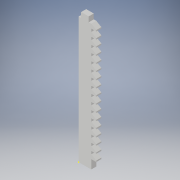
# Autodesk Inventor part: graduated_foot
Saved by Autodesk Inventor 2019.4 (Build 234330000, 330)
## iProperties
Created: 2019-12-14
Part Number: graduated_foot
Material: Generic
Document SubType Name: Modeling
Designer: fabfarm
Density: 1 g/cm^3
Appearance: Default
Author: fabfarm
Autodesk Inventor part; units mm, degrees
ref_plane "YZ Plane" through (0, 0, 0) normal (1, 0, 0) x (0, 1, 0)
ref_plane "XZ Plane" through (0, 0, 0) normal (0, 1, 0) x (-1, 0, 0)
ref_plane "XY Plane" through (0, 0, 0) normal (0, 0, 1) x (1, 0, 0)
sketch "Sketch4" plane through (0, 0, 0) normal (0, 0, 1) x (1, 0, 0)
  line L0 (0, 500) -> (50, 500)
  line L1 (50, 500) -> (50, 0)
  line L2 (50, 0) -> (0, 0)
  line L3 (0, 0) -> (0, 500)
  dimension "d31" = 50
  dimension "d32" = 500
  constraints: 8 end point, 2 parallel, 2 point on line, 1 horizontal, 1 perpendicular
  measures "d31" distance of L0.start L0.end
  measures "d32" distance of L2.end L0.start
extrude "Extrusion1" add sketch "Sketch4" along normal blind 20.18
sketch "Sketch5" plane through (0, 0, 20.18) normal (0, 0, 1) x (1, 0, 0)
  line L0 (50, 500) -> (0, 500) projected
  line L1 (10, 500) -> (40, 500)
  line L2 (40, 500) -> (40, 520.18)
  line L3 (40, 520.18) -> (10, 520.18)
  line L4 (10, 520.18) -> (10, 500)
  line L5 (0, 500) -> (0, 0) projected
  line L6 (50, 0) -> (50, 500) projected
  dimension "d46" = 10
  dimension "d47" = 10
  dimension "d48" = 20.18
  constraints: 8 end point, 2 parallel, 1 horizontal, 1 perpendicular, 1 point on line
  measures "d46" distance between parallel lines of L5 L4
  measures "d47" distance between parallel lines of L6 L2
  measures "d48" distance of L3.end L1.start
extrude "Extrusion2" add sketch "Sketch5" against normal blind 20.18
sketch "Sketch6" plane through (0, 0, 20.18) normal (0, 0, 1) x (1, 0, 0)
  line L0 (50, 500) -> (70, 488.453)
  line L1 (70, 488.453) -> (70, 483.453)
  line L2 (70, 483.453) -> (50, 483.453)
  line L3 (50, 500) -> (40, 500) projected
  line L4 (40, 500) -> (50, 500) projected
  line L5 (50, 500) -> (50, 483.453)
  line L6 (50, 0) -> (50, 500) projected
  line L7 (50, 472) -> (70, 460.453)
  line L8 (70, 460.453) -> (70, 455.453)
  line L9 (70, 455.453) -> (50, 455.453)
  line L10 (50, 472) -> (50, 455.453)
  line L11 (50, 444) -> (70, 432.453)
  line L12 (70, 432.453) -> (70, 427.453)
  line L13 (70, 427.453) -> (50, 427.453)
  line L14 (50, 444) -> (50, 427.453)
  line L15 (50, 416) -> (70, 404.453)
  line L16 (70, 404.453) -> (70, 399.453)
  line L17 (70, 399.453) -> (50, 399.453)
  line L18 (50, 416) -> (50, 399.453)
  line L19 (50, 388) -> (70, 376.453)
  line L20 (70, 376.453) -> (70, 371.453)
  line L21 (70, 371.453) -> (50, 371.453)
  line L22 (50, 388) -> (50, 371.453)
  line L23 (50, 360) -> (70, 348.453)
  line L24 (70, 348.453) -> (70, 343.453)
  line L25 (70, 343.453) -> (50, 343.453)
  line L26 (50, 360) -> (50, 343.453)
  line L27 (50, 332) -> (70, 320.453)
  line L28 (70, 320.453) -> (70, 315.453)
  line L29 (70, 315.453) -> (50, 315.453)
  line L30 (50, 332) -> (50, 315.453)
  line L31 (50, 304) -> (70, 292.453)
  line L32 (70, 292.453) -> (70, 287.453)
  line L33 (70, 287.453) -> (50, 287.453)
  line L34 (50, 304) -> (50, 287.453)
  line L35 (50, 276) -> (70, 264.453)
  line L36 (70, 264.453) -> (70, 259.453)
  line L37 (70, 259.453) -> (50, 259.453)
  line L38 (50, 276) -> (50, 259.453)
  line L39 (50, 248) -> (70, 236.453)
  line L40 (70, 236.453) -> (70, 231.453)
  line L41 (70, 231.453) -> (50, 231.453)
  line L42 (50, 248) -> (50, 231.453)
  line L43 (50, 220) -> (70, 208.453)
  line L44 (70, 208.453) -> (70, 203.453)
  line L45 (70, 203.453) -> (50, 203.453)
  line L46 (50, 220) -> (50, 203.453)
  line L47 (50, 192) -> (70, 180.453)
  line L48 (70, 180.453) -> (70, 175.453)
  line L49 (70, 175.453) -> (50, 175.453)
  line L50 (50, 192) -> (50, 175.453)
  line L51 (50, 164) -> (70, 152.453)
  line L52 (70, 152.453) -> (70, 147.453)
  line L53 (70, 147.453) -> (50, 147.453)
  line L54 (50, 164) -> (50, 147.453)
  line L55 (50, 136) -> (70, 124.453)
  line L56 (70, 124.453) -> (70, 119.453)
  line L57 (70, 119.453) -> (50, 119.453)
  line L58 (50, 136) -> (50, 119.453)
  line L59 (50, 108) -> (70, 96.453)
  line L60 (70, 96.453) -> (70, 91.453)
  line L61 (70, 91.453) -> (50, 91.453)
  line L62 (50, 108) -> (50, 91.453)
  line L63 (50, 80) -> (70, 68.453)
  line L64 (70, 68.453) -> (70, 63.453)
  line L65 (70, 63.453) -> (50, 63.453)
  line L66 (50, 80) -> (50, 63.453)
  line L67 (50, 52) -> (70, 40.453)
  line L68 (70, 40.453) -> (70, 35.453)
  line L69 (70, 35.453) -> (50, 35.453)
  line L70 (50, 52) -> (50, 35.453)
  line L71 (50, 24) -> (70, 12.453)
  line L72 (70, 12.453) -> (70, 7.453)
  line L73 (70, 7.453) -> (50, 7.453)
  line L74 (50, 24) -> (50, 7.453)
  point P0 (0, 0)
  point P1 (40, 472)
  point P2 (40, 444)
  point P3 (40, 416)
  point P4 (40, 388)
  point P5 (40, 360)
  point P6 (40, 332)
  point P7 (40, 304)
  point P8 (40, 276)
  point P9 (40, 248)
  point P10 (40, 220)
  point P11 (40, 192)
  point P12 (40, 164)
  point P13 (40, 136)
  point P14 (40, 108)
  point P15 (40, 80)
  point P16 (40, 52)
  point P17 (40, 24)
  dimension "d49" = 20
  dimension "d50" = 30
  dimension "d51" = 5
  dimension "d54" = 28
  constraints: 144 end point, 1 collinear, 1 horizontal, 1 perpendicular, 1 vertical, 153 other
  measures "d49" distance of L1.end L2.end
  measures "d50" angle of L3 L0
  measures "d51" distance of L0.end L1.end
  measures "d54" distance of L0.start L7.start
extrude "Extrusion3" add sketch "Sketch6" against normal blind 20.18 contours L0 L1 L2 L5 | L6 L67 L68 L69 | L6 L63 L64 L65 | L6 L59 L60 L61 | L6 L55 L56 L57 | L6 L51 L52 L53 | L6 L47 L48 L49 | L6 L43 L44 L45 | L6 L39 L40 L41 | L6 L35 L36 L37 | L6 L31 L32 L33 | L6 L27 L28 L29 | L6 L23 L24 L25 | L6 L19 L20 L21 | L6 L15 L16 L17 | L6 L11 L12 L13 | L6 L7 L8 L9
sketch "Sketch7" plane through (0, 0, 20.18) normal (0, 0, 1) x (1, 0, 0)
  point P0 (0, 0)
body "Solid1"
